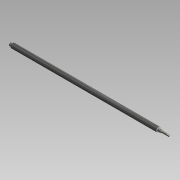
# Autodesk Inventor part: MTSBRK12-420-F7-R8-T9-Q8-S20-E5-FE0-FW7-FY1
Saved by Autodesk Inventor 2020.1 (Build 241239000, 239)
## iProperties
Created: 2019-12-03
Part Number: MTSBRK12-420-F7-R8-T9-Q8-S20-E5-FE0-FW7-FY1
Catalog Web Link: https://us.misumi-ec.com/vona2/detail/110302641830/?HissuCode=MTSBRK12-420-F7-R8-T9-Q8-S20-E5-FE0-FW7-FY1
Description: MTSRK, MTSBRK, RMTSRK, MTSLK, MTSBLK, RMTSLK, MTSWKA, MTSBWKA, RMTSWKA, MTSWKB, MTSBWKB, RMTSWKB-Lead Screws One End Stepped / One End Double Stepped Right-Hand Screw / Left-Hand Screw / Right and Left-Hand Screw 1045 Carbon Steel
Vendor: MISUMI
Document SubType Name: Modeling
Designer: psAdmin
Manufacturer: MISUMI
Mass: 350.139 g
Surface Area: 153.947 cm^2
Volume: 44.6037 cm^3
Density: 7.85 g/cm^3
Material: Steel, Carbon
Appearance: Semi-Polished
Category: FIRSTChoice
PSOL_IDENT_0: {$CADENAS_DATA\23d-libs\misumi\metric\10_lead_screws\mtsrk.prj},492 {VTYP=3D},{NB=MTSBRK12-420-F7-R8
PSOL_IDENT_1: -T9-Q8-S20-E5-FE0-FW7-FY1},{LINA=MTSBRK12-420-F7-R8-T9-Q8-S20-E5-FE0-FW7-FY1},{NN=MTSRK, MTSBRK, RMT
PSOL_IDENT_2: SRK, MTSLK, MTSBLK, RMTSLK, MTSWKA, MTSBWKA, RMTSWKA, MTSWKB, MTSBWKB, RMTSWKB},{DATE=17.06.2016 05:
PSOL_IDENT_3: 46:50},{GEOMDATE=16.10.2014 00:00:00},{VERSION=},{LINEID=10},{LINESUBID=-1},{WBVAR=THDS,TS,ST,L,F,G,
PSOL_IDENT_4: T,S,V,Q,R,E,X,ALT1,FE,FR,FW,FY,ALT3AR,AR,ALT3AE,AE,ALT2,SE,SR,SW,SY,ALT4MR,MR,ALT4ME,ME,ALT5BV,BV,AL
PSOL_IDENT_5: T5BQ,BQ,ALT5BR,BR,ALT6,WALT6,AALT6,ALT7,KQ,KV,KE,KR,CALT7}  {NB=MTSBRK12-420-F7-R8-T9-Q8-S20-E5-FE0-
PSOL_IDENT_6: FW7-FY1},{LINA=MTSBRK12-420-F7-R8-T9-Q8-S20-E5-FE0-FW7-FY1},{KT=DUMMY},{PN=MTSBRK12-420-F7-R8-T9-Q8-
PSOL_IDENT_7: S20-E5-FE0-FW7-FY1},{TYPE=MTSBRK},{THDS=RHS},{TS=},{TSALG= '','N/A' },{ST=BO},{STALG= '-','-' , 'BO'
PSOL_IDENT_8: ,'Black Oxide' , 'LTBCP','Low Temperature Black Chrome Plating' },{D=12},{L=420},{LMIN=80},{LMAX=100
PSOL_IDENT_9: 0},{F=7},{FALG=[2:45/1]},{FMIN=2},{FMAX=45},{FMAXRT=45},{FMAXLT=40},{G=0},{GALG=[0]},{GMIN=2},{GMAXL
PSOL_IDENT_10: T=45},{GPN=},{T=9},{TALG=[2:45/1]},{TMIN=2},{TMAX=45},{TMAXRT=45},{TPN=-T9},{S=20},{SALG=[2:40/1]},{
PSOL_IDENT_11: SMIN=2},{SMAX=40},{SMAXRT=40},{SMAXLT=45},{V=0},{VALG=0},{VS=[7,8,9]},{VPN=},{Q=8},{QALG=[7,8,9]},{Q
PSOL_IDENT_12: S=[7,8,9]},{QPN=-Q8},{R=8},{RALG=[7,8,9]},{RS1=[7,8,9]},{RS2=[7,8,9]},{E=5},{EALG=[4:7/1]},{EMINQ=4}
PSOL_IDENT_13: ,{EMINQ1=4},{EMINQ2=4},{EMAXQ=7},{EMINV=-1},{EMINV1=2},{EMINV2=0},{EMAXV=-1},{X=0},{XALG=[0]},{XMIN=
PSOL_IDENT_14: 0},{XMAX=0},{XPN=},{Y=0},{YMAX=431},{YMIN=22},{D2=12},{P=2},{ALT1=FE},{ALT1ALG= '','w/o Flat Machini
PSOL_IDENT_15: ng' , 'FE','with FE (Flat Machining)' , 'FR','with FR (Flat Machining)' },{FE=0},{FEALG=[0],[2:15/0.
PSOL_IDENT_16: 5]},{FEMAX=15},{FR=0},{FRALG=[0]},{FRMAX=2},{FW=7},{FWALG=[3:18/0.5]},{FWMAX=18},{FY=1},{FYALG=[0.5:
PSOL_IDENT_17: 1/0.5]},{FYMAX=1},{ALT1PN=-FE0-FW7-FY1},{ALT3AR=},{ALT3ARALG= '','w/o AR (Retaining Ring Groove)' , '
PSOL_IDENT_18: AR','with AR (Retaining Ring Groove)' },{AR=0.0},{ARALG=[0]},{ARMIN=2},{ARMAX=4.9},{AREE=5},{ARNN=1.
PSOL_IDENT_19: 2},{ARMM=0.84},{EEALT3AR=0.0},{MMALT3AR=0.00},{NNALT3AR=0.0},{ARPN=-AR0.0},{ALT3AE=},{ALT3AEALG= '','
PSOL_IDENT_20: Not applicable' },{AE=0.0},{AEALG=[0]},{AEMIN=11},{AEMAX=28.9},{AEEE=0},{AENN=0},{AEMM=0},{EEALT3AE=
PSOL_IDENT_21: 0.0},{MMALT3AE=0.00},{NNALT3AE=0.0},{AEPN=-AE0.0},{ALT3PN=},{ALT2=},{ALT2ALG= '','w/o Wrench Flats'
PSOL_IDENT_22: , 'SE','with SE (Wrench Flats)' , 'SR','with SR (Wrench Flats)' },{SE=0},{SEALG=[0]},{SEMAX=15},{SR=
PSOL_IDENT_23: 0},{SRALG=[0]},{SRMAX=2},{SW=0},{SWALG=[0]},{SWMIN=0},{SWMAX=0},{SY=0},{SYALG=[0]},{SYMAX=0},{ALT2PN=
PSOL_IDENT_24: },{ALT4MR=},{ALT4MRALG= '','w/o MR (Coarse Tapping)' , 'MR','with MR (Coarse Tapping)' },{MR=0},{MRA
PSOL_IDENT_25: LG=[0]},{PALT4MR=0},{ALT4ME=},{ALT4MEALG= '','w/o ME (Coarse Tapping)' , 'ME','with ME (Coarse Tappi
PSOL_IDENT_26: ng)' },{ME=0},{MEALG=[0]},{PALT4ME=0},{ALT4PN=},{ALT5BV=},{ALT5BVALG= '','Not applicable' },{BV=0},{
PSOL_IDENT_27: BVALG=[0]},{BVMIN=3},{BVMAX=-3},{MALT5BV=0},{PALT5BV=1},{MPALT5BV=0},{ALT5BQ=},{ALT5BQALG= '','w/o B
PSOL_IDENT_28: Q (Threaded)' , 'BQ','with BQ (Threaded)' },{BQ=0},{BQALG=[0]},{BQMIN=3},{BQMAX=6},{MALT5BQ=8},{PALT
PSOL_IDENT_29: 5BQ=1},{MPALT5BQ=0},{ALT5BR=},{ALT5BRALG= '','w/o BR (Threaded)' , 'BR','with BR (Threaded)' },{BR=0
PSOL_IDENT_30: },{BRALG=[0]},{BRMIN=3},{BRMAX=4},{MALT5BR=8},{PALT5BR=1},{DALT5BR=0},{MPALT5BR=0},{ALT5PN=},{ALT6=}
PSOL_IDENT_31: ,{ALT6ALG= '','w/o Square Chamfering' , 'ZR','with ZR (Square Chamfering)' },{ZR=0},{ZE=0},{WALT6=0}
PSOL_IDENT_32: ,{WALT6ALG=0},{WALT6ZR=[0]},{WALT6ZE=[0]},{WALT6ZRMIN=0},{WALT6ZEMIN=0},{WALT6ZRMAX=-1},{WALT6ZEMAX=
PSOL_IDENT_33: -1},{AALT6=0},{AALT6ALG=[0]},{AALT6MAXF=5},{AALT6MAXS=18},{ALT6PN=},{ALT7=},{ALT7ALG= '','w/o Keyway'
PSOL_IDENT_34: , 'KQ','with KQ (Keyway)' , 'KR','with KR (Keyway)' },{KQ=0},{KQALG=[0]},{KQMAX=4},{KV=0},{KVALG=[0
PSOL_IDENT_35: ]},{KVMAX=-4},{KE=0},{KEALG=[0]},{KEMAX=16},{KR=0},{KRALG=[0]},{KRMAX=2},{CALT7=0},{CALT7ALG=[0]},{C
PSOL_IDENT_36: ALT7MIN=0},{CLAT7MAX=0},{BB1ALT7KQ=3},{BB1ALT7KV=2},{BB1ALT7KE=2},{BB1ALT7KR=3},{BB1ALT7=0},{TT1ALT7
PSOL_IDENT_37: KQ=1.8},{TT1ALT7KV=1.2},{TT1ALT7KE=1.2},{TT1ALT7KR=1.8},{TT1ALT7=0.0},{ALT7PN=},{ERRORPN=},{ERRORALT
PSOL_IDENT_38: 12=OK},{ERRORALT13=OK},{ERRORALT14=OK},{ERRORALT15=OK},{ERRORALT17=OK},{ERRORALT23=OK},{ERRORALT24=O
PSOL_IDENT_39: K},{ERRORALT25=OK},{ERRORALT27=OK},{ERRORALT34=OK},{ERRORALT35=OK},{ERRORALT37=OK},{ERRORALT45=OK},{
PSOL_IDENT_40: ERRORALT46=OK},{ERRORALT47=OK},{ERRORALT57=OK},{ERRORALT67=OK}
NN: MTSRK, MTSBRK, RMTSRK, MTSLK, MTSBLK, RMTSLK, MTSWKA, MTSBWKA, RMTSWKA, MTSWKB, MTSBWKB, RMTSWKB
NT: Lead Screws One End Stepped / One End Double Stepped Right-Hand Screw / Left-Hand Screw / Right and Left-Hand Screw 1045 Carbon Steel
NB: MTSBRK12-420-F7-R8-T9-Q8-S20-E5-FE0-FW7-FY1
NBSYN: $PN.
LINA: MTSBRK12-420-F7-R8-T9-Q8-S20-E5-FE0-FW7-FY1
PN: MTSBRK12-420-F7-R8-T9-Q8-S20-E5-FE0-FW7-FY1
THDS: Right-Hand Screw
TS: N/A
ST: Black Oxide
D: 12
L: 420
F: 7
G: 0
T: 9
S: 20
V: 0
Q: 8
R: 8
E: 5
X: 0
D2: 12
P: 2
ALT1: with FE (Flat Machining)
FE: 0
FR: 0
FW: 7
FY: 1
ALT3AR: w/o AR (Retaining Ring Groove)
AR: 0.0
EEALT3AR: 0.0
MMALT3AR: 0.00
NNALT3AR: 0.0
ALT3AE: Not applicable
AE: 0.0
EEALT3AE: 0.0
MMALT3AE: 0.00
NNALT3AE: 0.0
ALT2: w/o Wrench Flats
SE: 0
SR: 0
SW: 0
SY: 0
ALT4MR: w/o MR (Coarse Tapping)
MR: 0
ALT4ME: w/o ME (Coarse Tapping)
ME: 0
ALT5BV: Not applicable
BV: 0
MPALT5BV: 0
ALT5BQ: w/o BQ (Threaded)
BQ: 0
MPALT5BQ: 0
ALT5BR: w/o BR (Threaded)
BR: 0
MPALT5BR: 0
ALT6: w/o Square Chamfering
WALT6: 0
AALT6: 0
ALT7: w/o Keyway
KQ: 0
KV: 0
KE: 0
KR: 0
CALT7: 0
BB1ALT7: 0
TT1ALT7: 0.0
SUPPLIER: MISUMI
ARTICLENO: MTSBRK12-420-F7-R8-T9-Q8-S20-E5-FE0-FW7-FY1
BOMINFO: MTSBRK12-420-F7-R8-T9-Q8-S20-E5-FE0-FW7-FY1
CREATOR: CADENAS GmbH
Author: Autodesk Inc.
Comments: Lead Screws One End Stepped / One End Double Stepped Right-Hand Screw / Left-Hand Screw / Right and Left-Hand Screw 1045 Carbon Steel
Autodesk Inventor part; units mm, degrees
ref_plane "YZ Plane" through (0, 0, 0) normal (1, 0, 0) x (0, 1, 0)
ref_plane "XZ Plane" through (0, 0, 0) normal (0, 1, 0) x (-1, 0, 0)
ref_plane "XY Plane" through (0, 0, 0) normal (0, 0, 1) x (1, 0, 0)
sketch "Sketch_16" plane through (0, 0, 0) normal (0, 0, 1) x (1, 0, 0)
  line L0 (391, 0) -> (7, 0)
  line L1 (7, 0) -> (7, 6)
  line L2 (7, 6) -> (391, 6)
  line L3 (391, 6) -> (391, 0)
  line L4 (391, 0) -> (7, 0)
  constraints: 10 end point
revolve "Revolution1" add sketch "Sketch_16" angle 360 about axis through (391, 0, 0) along (1, 0, 0)
thread "Thread1" size "TR12x2" class "7e" standard "ISO Metric Trapezoidal Threads" full length
sketch "Sketch_23" plane through (0, 0, 0) normal (0, 0, 1) x (1, 0, 0)
  line L0 (7, 0) -> (0, 0)
  line L1 (0, 0) -> (0, 3.5)
  line L2 (0, 3.5) -> (0.5, 4)
  line L3 (0.5, 4) -> (6.7, 4)
  arc A0 (6.7, 4) -> (7, 4.3) centre (6.7, 4.3) ccw
  line L4 (7, 4.3) -> (7, 0)
  line L5 (7, 0) -> (0, 0)
  constraints: 12 end point, 2 point on circle, 1 centre point
revolve "Revolution2" add sketch "Sketch_23" angle 360 about axis through (7, 0, 0) along (1, 0, 0)
sketch "Sketch_4" plane through (0, 0, 0) normal (0, 0, 1) x (1, 0, 0)
  line L0 (420, 0) -> (391, 0)
  line L1 (391, 0) -> (391, 4.3)
  arc A0 (391, 4.3) -> (391.3, 4) centre (391.3, 4.3) ccw
  line L2 (391.3, 4) -> (400, 4)
  line L3 (400, 4) -> (400, 2.8)
  arc A1 (400, 2.8) -> (400.3, 2.5) centre (400.3, 2.8) ccw
  line L4 (400.3, 2.5) -> (419.5, 2.5)
  line L5 (419.5, 2.5) -> (420, 2)
  line L6 (420, 2) -> (420, 0)
  line L7 (420, 0) -> (391, 0)
  constraints: 16 end point, 4 point on circle, 2 centre point
revolve "Revolution3" add sketch "Sketch_4" angle 360 about axis through (420, 0, 0) along (1, 0, 0)
sketch "Sketch_8" plane through (420, 0, 0) normal (1, 0, 0) x (0, 0, -1)
  line L0 (-2.5, -6) -> (-1.5, -6)
  line L1 (-1.5, -6) -> (-1.5, 6)
  line L2 (-1.5, 6) -> (-2.5, 6)
  line L3 (-2.5, 6) -> (-2.5, -6)
  constraints: 8 end point
extrude "Extrusion1" cut sketch "Sketch_8" against normal blind 7
body "Solid1"
